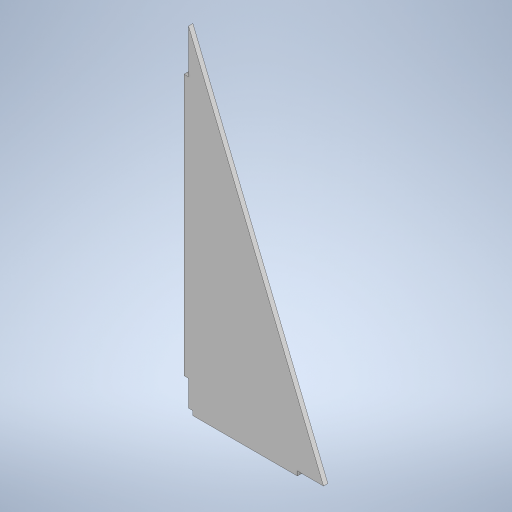
# Autodesk Inventor part: side support
Saved by Autodesk Inventor 2023 (Build 270158000, 158)
## iProperties
Created: 2023-10-15
Part Number: side support
Material: Generic
Document SubType Name: Modeling
Designer: Nate
Density: 1 g/cm^3
Appearance: Default
Author: Nate
Autodesk Inventor part; units mm, degrees
ref_plane "YZ Plane" through (0, 0, 0) normal (1, 0, 0) x (0, 1, 0)
ref_plane "XZ Plane" through (0, 0, 0) normal (0, 1, 0) x (-1, 0, 0)
ref_plane "XY Plane" through (0, 0, 0) normal (0, 0, 1) x (1, 0, 0)
sketch "Sketch1" plane through (0, 0, 0) normal (0, 0, 1) x (1, 0, 0)
  line L0 (0, 0) -> (152.4, 0)
  line L1 (152.4, 0) -> (152.4, 6.35)
  line L2 (152.4, 6.35) -> (0, 6.35)
  line L3 (0, 6.35) -> (0, 0)
  line L4 (0, 6.35) -> (6.35, 6.35)
  line L5 (152.4, 6.35) -> (190.5, 6.35)
  line L6 (0, 6.35) -> (6.35, 6.35)
  line L7 (-6.35, 425.45) -> (0, 425.45)
  line L8 (0, 6.35) -> (-6.35, 6.35)
  line L9 (-6.35, 6.35) -> (-6.35, 488.95)
  line L10 (-6.35, 488.95) -> (0, 488.95)
  line L11 (0, 488.95) -> (0, 6.35)
  line L12 (-6.35, 43.9506) -> (-12.7, 43.9506)
  line L13 (-12.7, 43.9506) -> (-12.7, 424.9506)
  line L14 (-12.7, 424.9506) -> (-6.35, 424.9506)
  line L15 (-6.35, 424.9506) -> (-6.35, 43.9506)
  line L16 (190.5, 6.35) -> (-6.35, 488.95)
  point P0 (3.175, 6.35)
  point P1 (-3.175, 6.35)
  point P2 (-9.525, 43.9506)
  dimension "d0" = 152.4
  dimension "d1" = 6.35
  dimension "d7" = 38.1
  dimension "d12" = 6.35
  dimension "d15" = 6.35
  dimension "d16" = 482.6
  dimension "d17" = 6.35
  dimension "d18" = 381
  dimension "d19" = 37.6006
  constraints: 34 end point, 6 horizontal, 6 parallel, 3 midpoint, 3 perpendicular, 1 point on line
  measures "d0" distance of L2.end L1.end
  measures "d1" distance of L1.end L0.end
  measures "d7" distance of L1.end L5.end
  measures "d12" distance of L7.start L7.end
  measures "d15" distance between parallel lines of L11 L9
  measures "d16" distance from line of point (-3.175, 6.35) L10
  measures "d17" distance of L13.end L14.end
  measures "d18" distance of L12.end L13.end
  measures "d19" distance from line of L2 point (-9.525, 43.951)
extrude "Extrusion1" add sketch "Sketch1" along normal blind 6.35 contours L3 L2 L1 L0 | L11 L16 L5 L2 | L8 L9 L7 L11 | L7 L9 L16 L11 | L12 L13 L14 L9
body "Solid1"
